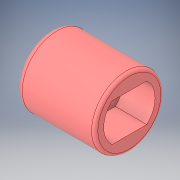
# Autodesk Inventor part: servo_adapter
Saved by Autodesk Inventor 2019 (Build 230136000, 136)
## iProperties
Created: 2019-01-24
Part Number: servo_adapter
Material: Generic
Document SubType Name: Modeling
Designer: assman
Density: 1 g/cm^3
Appearance: PET Pink
Author: assman
## iProperties of the stored document servo_adapter_3DPrint.ipt
Created: 2019-01-24
Part Number: servo_adapter_3DPrint
Material: Generic
Document SubType Name: Modeling
Designer: assman
Density: 1 g/cm^3
Appearance: Default
Author: assman
Autodesk Inventor part; units mm, degrees
ref_plane "YZ Plane" through (0, 0, 0) normal (1, 0, 0) x (0, 1, 0)
ref_plane "XZ Plane" through (0, 0, 0) normal (0, 1, 0) x (-1, 0, 0)
ref_plane "XY Plane" through (0, 0, 0) normal (0, 0, 1) x (1, 0, 0)
sketch "Sketch5" plane through (0, 0, 0) normal (1, 0, 0) x (0, 1, 0)
  circle A0 centre (0, 0) radius 5.5
  dimension "d11" = 11
  constraints: 1 centre point, 1 coincident
  measures "d11" diameter of A0
extrude "Extrusion5" add sketch "Sketch5" along normal blind 4
sketch "Sketch7" plane through (4, 0, 0) normal (1, 0, 0) x (0, 0, -1)
  circle A0 centre (0, 0) radius 5.5 projected
  constraints: 1 coincident
hole "Hole1" at (4, 0, 0) direction (-1, 0, 0) diameter 3.121 end through all counterbore diameter 5.3 counterbore depth 2.4
sketch "Sketch10" plane through (4, 0, 0) normal (1, 0, 0) x (0, 0, -1)
  line L0 (-2.7575, 3.0003) -> (2.7575, 3.0003)
  line L1 (2.7575, -3.0003) -> (-2.7575, -3.0003)
  line L2 (-2.7575, 3.0003) -> (2.7575, -3.0003) construction
  line L3 (2.7575, 3.0003) -> (-2.7575, -3.0003) construction
  arc A0 (2.7575, 3.0003) -> (-2.7575, 3.0003) centre (0, 0) ccw
  arc A1 (-2.7575, -3.0003) -> (2.7575, -3.0003) centre (0, 0) ccw
  constraints: 8 end point, 4 point on circle, 2 centre point, 2 midpoint, 1 horizontal, 1 parallel
extrude "Extrusion8" add sketch "Sketch10" along normal blind 5
sketch "Sketch11" plane through (4, 0, 0) normal (1, 0, 0) x (0, 0, -1)
  circle A0 centre (0, 0) radius 1.5605 projected
  circle A1 centre (0, 0) radius 4.075
  circle A2 centre (0, 0) radius 5.5 projected
  constraints: 1 centre point
sketch "Sketch12" plane through (0, 0, 0) normal (-1, 0, 0) x (0, 0, 1)
  circle A0 centre (0, 0) radius 2.975
  circle A1 centre (0, 0) radius 5.5 projected
  dimension "d35" = 5.95
  constraints: 1 centre point, 1 coincident
  measures "d35" diameter of A0
extrude "Extrusion10" add sketch "Sketch12" along normal blind 3.5
extrude "Extrusion11" add sketch "Sketch11" along normal blind 5 contours A2
fillet "Fillet4" radius 1 1 edges at (-3.5, 0, -5.5)
fillet "Fillet4" radius 0.5 1 edges at (9, 0, 5.5)
body "Solid1"
body "Solid2"
